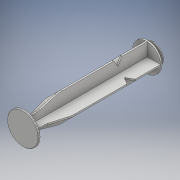
# Autodesk Inventor part: Jeringa core
Saved by Autodesk Inventor 2018.3 (Build 223284000, 284)
## iProperties
Created: 2019-02-24
Part Number: Jeringa core
Material: Generic
Document SubType Name: Modeling
Designer: Mario
Density: 1 g/cm^3
Appearance: Default
Author: Mario
Autodesk Inventor part; units mm, degrees
sketch "Sketch1" plane through (0, 0, 0) normal (0, 1, 0) x (-1, 0, 0)
  line L0 (0.75, 0.75) -> (13.75, 0.75)
  line L1 (13.75, 0.75) -> (13.75, -0.75)
  line L2 (13.75, -0.75) -> (0.75, -0.75)
  line L3 (0.75, -0.75) -> (0.75, -13.75)
  line L4 (0.75, -13.75) -> (-0.75, -13.75)
  line L5 (-0.75, -13.75) -> (-0.75, -0.75)
  line L6 (-0.75, -0.75) -> (-13.75, -0.75)
  line L7 (-13.75, -0.75) -> (-13.75, 0.75)
  line L8 (-13.75, 0.75) -> (-0.75, 0.75)
  line L9 (-0.75, 0.75) -> (-0.75, 13.75)
  line L10 (-0.75, 13.75) -> (0.75, 13.75)
  line L11 (0.75, 13.75) -> (0.75, 0.75)
  line L12 (0.75, 0.75) -> (-0.75, -0.75) construction
  line L13 (-0.75, 0.75) -> (0.75, -0.75) construction
  point P0 (0, 0)
  point P1 (0, 0)
  dimension "d0" = 1.5
  dimension "d24" = 27.5
  constraints: 28 end point, 10 perpendicular, 5 equal length, 5 point on line, 1 coincident, 1 midpoint, 1 vertical
  measures "d0" distance of L6.end L7.end
  measures "d24" distance between parallel lines of L7 L1
extrude "Extrusion1" add sketch "Sketch1" along normal blind 25
sketch "Sketch2" plane through (0, 25, 0) normal (0, 1, 0) x (1, 0, 0)
  circle A0 centre (0, 0) radius 13.75
  dimension "d4" = 27.5
  constraints: 1 centre point, 1 coincident
  measures "d4" diameter of A0
extrude "Extrusion2" add sketch "Sketch2" along normal blind 1.5
sketch "Sketch3" plane through (0, 26.5, 0) normal (0, 1, 0) x (1, 0, 0)
  line L0 (-0.75, -0.75) -> (-7.25, -0.75)
  line L1 (-0.75, -0.75) -> (-13.75, -0.75) projected
  line L2 (-7.25, 0.75) -> (-0.75, 0.75)
  line L3 (0.75, 0.75) -> (7.25, 0.75)
  line L4 (0.75, 0.75) -> (13.75, 0.75) projected
  line L5 (7.25, 0.75) -> (7.25, -0.75)
  line L6 (7.25, -0.75) -> (0.75, -0.75)
  line L7 (0.75, -0.75) -> (0.75, -7.75)
  line L8 (0.75, -7.75) -> (-0.75, -7.75)
  line L9 (-0.75, -13.75) -> (-0.75, -0.75) projected
  line L10 (-0.75, -7.75) -> (-0.75, -0.75)
  line L11 (-0.75, -0.75) -> (-0.75, 0.75)
  line L12 (-0.75, 7.75) -> (0.75, 7.75)
  line L13 (0.75, 7.75) -> (0.75, 0.75)
  line L14 (-0.75, 0.75) -> (-0.75, 13.75) projected
  line L15 (-0.75, 0.75) -> (-0.75, 7.75)
  line L16 (-7.25, 0.75) -> (-7.25, -0.75)
  dimension "d48" = 15.5
  constraints: 26 end point, 6 perpendicular, 2 collinear, 2 equal length, 2 midpoint, 2 point on line, 1 horizontal, 1 parallel, 1 vertical
  measures "d48" distance between parallel lines of L12 L8
extrude "Extrusion3" add sketch "Sketch3" along normal blind 4
sketch "Sketch4" plane through (0, 30.5, 0) normal (0, 1, 0) x (1, 0, 0)
  circle A0 centre (0, 0) radius 13.75 construction
  arc A1 (13.72953, 0.75) -> (0.75, 13.72953) centre (0, 0) ccw construction
  arc A2 (13.72953, -0.75) -> (13.75, 0) centre (0, 0) ccw
  arc A3 (13.75, 0) -> (13.72953, 0.75) centre (0, 0) ccw
  arc A4 (0.75, 13.72953) -> (0, 13.75) centre (0, 0) ccw construction
  arc A5 (0, 13.75) -> (-0.75, 13.72953) centre (0, 0) ccw
  arc A6 (-0.75, 13.72953) -> (-13.72953, 0.75) centre (0, 0) ccw construction
  arc A7 (-13.72953, 0.75) -> (-13.75, 0) centre (0, 0) ccw construction
  arc A8 (-13.75, 0) -> (-13.72953, -0.75) centre (0, 0) ccw construction
  arc A9 (-13.72953, -0.75) -> (-0.75, -13.72953) centre (0, 0) ccw construction
  arc A10 (-0.75, -13.72953) -> (0, -13.75) centre (0, 0) ccw construction
  arc A11 (0, -13.75) -> (0.75, -13.72953) centre (0, 0) ccw construction
  arc A12 (0.75, -13.72953) -> (13.72953, -0.75) centre (0, 0) ccw construction
  circle A13 centre (0, 0) radius 10.25
  dimension "d50" = 20.5
  constraints: 1 centre point, 1 coincident
  measures "d50" diameter of A13
extrude "Extrusion4" add sketch "Sketch4" along normal blind 1
ref_plane "Work Plane1" through (0, -4, 0) normal (0, -1, 0) x (1, 0, 0)
sketch "Sketch6" plane through (0, -4, 0) normal (0, -1, 0) x (1, 0, 0)
  line L0 (0.75, 0.75) -> (6.75, 0.75)
  line L1 (0.75, -0.75) -> (6.75, -0.75)
  line L2 (6.75, 0.75) -> (6.75, -0.75)
  line L3 (0.75, -0.75) -> (0.75, -6.75)
  line L4 (0.75, -6.75) -> (-0.75, -6.75)
  line L5 (-0.75, -6.75) -> (-0.75, -0.75)
  line L6 (-0.75, -0.75) -> (-6.75, -0.75)
  line L7 (-6.75, -0.75) -> (-6.75, 0.75)
  line L8 (-6.75, 0.75) -> (-0.75, 0.75)
  line L9 (-0.75, 0.75) -> (-0.75, 6.75)
  line L10 (-0.75, 6.75) -> (0.75, 6.75)
  line L11 (0.75, 6.75) -> (0.75, 0.75)
  point P0 (0, 0)
  dimension "d17" = 13.5
  constraints: 24 end point, 7 perpendicular, 3 equal length, 2 point on line, 2 vertical, 1 horizontal, 1 parallel
  measures "d17" distance of L0.end L7.end
loft "Loft1" add profiles "Sketch6" section 1 edges at (-7.25, 0, 0.75) (-13.75, 0, 0) (-7.25, 0, -0.75) (-0.75, 0, -7.25) (0, 0, -13.75) (0.75, 0, -7.25) (7.25, 0, -0.75) (13.75, 0, 0) (7.25, 0, 0.75) (0.75, 0, 7.25) (0, 0, 13.75) (-0.75, 0, 7.25)
ref_plane "Work Plane2" through (-6.75, -8, 0.75) normal (0, -1, 0) x (1, 0, 0)
sketch "Sketch7" plane through (-6.75, -8, 0.75) normal (0, -1, 0) x (1, 0, 0)
  line L0 (7.5, 0) -> (20.47953, 0)
  line L1 (7.5, 0) -> (13.5, 0)
  line L2 (20.5, 0) -> (13.5, 0)
  line L3 (-6.97953, 0) -> (6, 0)
  line L4 (-7, 0) -> (0, 0)
  line L5 (0, 0) -> (6, 0)
  line L6 (6, 0) -> (6, 12.97953)
  line L7 (6, 0) -> (6, 6)
  line L8 (6, 13) -> (6, 6)
  line L9 (6, -14.47953) -> (6, -1.5)
  line L10 (6, -14.5) -> (6, -7.5)
  line L11 (6, -7.5) -> (6, -1.5)
  line L12 (7.5, 12.97953) -> (7.5, 0)
  line L13 (7.5, 13) -> (7.5, 6)
  line L14 (7.5, 6) -> (7.5, 0)
  line L15 (7.5, -1.5) -> (7.5, -14.47953)
  line L16 (7.5, -1.5) -> (7.5, -7.5)
  line L17 (7.5, -14.5) -> (7.5, -7.5)
  line L18 (20.5, -1.5) -> (20.5, 0)
  line L19 (7.5, 13) -> (6, 13)
  line L20 (-7, 0) -> (-7, -1.5)
  line L21 (6, -1.5) -> (-6.97953, -1.5)
  line L22 (6, -1.5) -> (0, -1.5)
  line L23 (-7, -1.5) -> (0, -1.5)
  line L24 (20.5, 0) -> (7.5, 0)
  line L25 (20.47953, -1.5) -> (7.5, -1.5)
  line L26 (20.5, -1.5) -> (13.5, -1.5)
  line L27 (13.5, -1.5) -> (7.5, -1.5)
  line L28 (6, -14.5) -> (7.5, -14.5)
  line L29 (6, -14.5) -> (6, -1.5)
  line L30 (-7, -1.5) -> (-7, 0)
  line L31 (-7, 0) -> (6, 0)
  line L32 (6, 13) -> (7.5, 13)
  line L33 (7.5, 0) -> (20.5, 0)
  line L34 (20.5, 0) -> (20.5, -1.5)
  line L35 (13.5, -1.5) -> (7.5, -1.5)
  line L36 (7.5, -1.5) -> (20.5, -1.5)
  line L37 (7.5, -14.5) -> (7.5, -1.5)
  line L38 (7.5, 0) -> (7.5, 13)
  line L39 (7.5, -14.5) -> (6, -14.5)
  line L40 (-7, -1.5) -> (6, -1.5)
  line L41 (6, 0) -> (6, 13)
  line L42 (6.75, -14.5) -> (6, -14.5)
  line L43 (7.5, -14.5) -> (6.75, -14.5)
  line L44 (20.5, -1.5) -> (20.47953, -1.5)
  line L45 (-6.97953, -1.5) -> (-7, -1.5)
  line L46 (-7, -0.75) -> (-7, 0)
  line L47 (-7, -1.5) -> (-7, -0.75)
  line L48 (6.75, 13) -> (7.5, 13)
  line L49 (6, 13) -> (6.75, 13)
  line L50 (20.5, -0.75) -> (20.5, -1.5)
  line L51 (20.5, 0) -> (20.5, -0.75)
  line L52 (7.5, -14.47953) -> (7.5, -14.5)
  line L53 (7.5, 13) -> (7.5, 12.97953)
  line L54 (6, -14.5) -> (6, -14.47953)
  line L55 (6, 12.97953) -> (6, 13)
  line L56 (-7, 0) -> (-6.97953, 0)
  line L57 (20.47953, 0) -> (20.5, 0)
  point P0 (6.75, -0.75)
  constraints: 24 end point, 5 perpendicular, 3 collinear, 2 parallel, 2 vertical, 2 other
sketch "Sketch7 outline for Loft2" plane through (-6.75, -8, 0.75) normal (0, -1, 0) x (1, 0, 0)
  line L0 (20.5, -1.5) -> (20.5, 0)
  line L1 (7.5, -1.5) -> (20.5, -1.5)
  line L2 (7.5, -14.5) -> (7.5, -1.5)
  line L3 (6, -14.5) -> (7.5, -14.5)
  line L4 (6, -1.5) -> (6, -14.5)
  line L5 (-7, -1.5) -> (6, -1.5)
  line L6 (-7, 0) -> (-7, -1.5)
  line L7 (6, 0) -> (-7, 0)
  line L8 (6, 13) -> (6, 0)
  line L9 (7.5, 13) -> (6, 13)
  line L10 (7.5, 0) -> (7.5, 13)
  line L11 (20.5, 0) -> (7.5, 0)
loft "Loft2" add profiles "Sketch7 outline for Loft2" section 1 edges at (-3.75, -4, 0.75) (-6.75, -4, 0) (-3.75, -4, -0.75) (-0.75, -4, -3.75) (0, -4, -6.75) (0.75, -4, -3.75) (3.75, -4, -0.75) (6.75, -4, 0) (3.75, -4, 0.75) (0.75, -4, 3.75) (0, -4, 6.75) (-0.75, -4, 3.75)
fillet "Fillet1" radius 0.5 8 edges at (0, -4, 6.75) (0, 0, 13.75) (-6.75, -4, 0) (-13.75, 0, 0) (0, -4, -6.75) (0, 0, -13.75) (6.75, -4, 0) (13.75, 0, 0)
sketch "Sketch8" plane through (-13.75, -8, -0.75) normal (0, -1, 0) x (1, 0, 0)
  line L0 (0, 1.5) -> (0, 0) projected
  line L1 (0, 0) -> (13, 0) projected
  line L2 (13, 0) -> (13, -13) projected
  line L3 (13, -13) -> (14.5, -13) projected
  line L4 (14.5, -13) -> (14.5, 0) projected
  line L5 (14.5, 0) -> (27.5, 0) projected
  line L6 (27.5, 0) -> (27.5, 1.5) projected
  line L7 (27.5, 1.5) -> (14.5, 1.5) projected
  line L8 (14.5, 1.5) -> (14.5, 14.5) projected
  line L9 (14.5, 14.5) -> (13, 14.5) projected
  line L10 (13, 14.5) -> (13, 1.5) projected
  line L11 (13, 1.5) -> (0, 1.5) projected
  point P0 (13.75, 0.75)
extrude "Extrusion5" add sketch "Sketch8" along normal blind 54
fillet "Fillet2" radius 0.5 4 edges at (0, -8, 13.75) (13.75, -8, 0) (0, -8, -13.75) (-13.75, -8, 0)
ref_plane "Work Plane3" through (-13.75, -82, -0.75) normal (0, -1, 0) x (1, 0, 0)
sketch "Sketch9" plane through (-13.75, -82, -0.75) normal (0, -1, 0) x (1, 0, 0)
  line L0 (14.5, 1.5) -> (21.75, 1.5)
  line L1 (21.75, 1.5) -> (21.75, 0)
  line L2 (21.75, 0) -> (14.5, 0)
  line L3 (14.5, 0) -> (14.5, -7.25)
  line L4 (14.5, -7.25) -> (13, -7.25)
  line L5 (13, -7.25) -> (13, 0)
  line L6 (13, 0) -> (5.75, 0)
  line L7 (5.75, 0) -> (5.75, 1.5)
  line L8 (5.75, 1.5) -> (13, 1.5)
  line L9 (13, 1.5) -> (13, 8.75)
  line L10 (13, 8.75) -> (14.5, 8.75)
  line L11 (14.5, 8.75) -> (14.5, 1.5)
  point P0 (13.75, 0.75)
  dimension "d29" = 16
  constraints: 24 end point, 7 parallel, 6 equal length, 3 perpendicular
  measures "d29" distance between parallel lines of L4 L10
loft "Loft3" add profiles "Sketch9" section 1 edges at (-13.75, -62, 0) (-7.25, -62, -0.75) (-0.75, -62, -7.25) (0, -62, -13.75) (0.75, -62, -7.25) (7.25, -62, -0.75) (13.75, -62, 0) (7.25, -62, 0.75) (0.75, -62, 7.25) (0, -62, 13.75) (-0.75, -62, 7.25) (-7.25, -62, 0.75)
sketch "Sketch10" plane through (-8, -82, -0.75) normal (0, -1, 0) x (1, 0, 0)
  line L0 (0, 0) -> (0, 1.5) projected
  line L1 (7.25, 0) -> (0, 0) projected
  line L2 (7.25, -7.25) -> (7.25, 0) projected
  line L3 (8.75, -7.25) -> (7.25, -7.25) projected
  line L4 (8.75, 0) -> (8.75, -7.25) projected
  line L5 (16, 0) -> (8.75, 0) projected
  line L6 (16, 1.5) -> (16, 0) projected
  line L7 (8.75, 1.5) -> (16, 1.5) projected
  line L8 (8.75, 8.75) -> (8.75, 1.5) projected
  line L9 (7.25, 8.75) -> (8.75, 8.75) projected
  line L10 (7.25, 1.5) -> (7.25, 8.75) projected
  line L11 (0, 1.5) -> (7.25, 1.5) projected
  point P0 (8, 0.75)
extrude "Extrusion6" add sketch "Sketch10" along normal blind 13
sketch "Sketch11" plane through (-8, -95, -0.75) normal (0, -1, 0) x (1, 0, 0)
  circle A0 centre (8, 0.75) radius 15.5
  dimension "d36" = 31
  constraints: 1 centre point, 1 coincident
  measures "d36" diameter of A0
extrude "Extrusion7" add sketch "Sketch11" along normal blind 2
fillet "Fillet3" radius 0.5 2 edges at (-15.5, -97, 0) (-15.5, -95, 0)
fillet "Fillet4" radius 10 4 edges at (0, -82, -8) (8, -82, 0) (0, -82, 8) (-8, -82, 0)
fillet "Fillet5" radius 20 4 edges at (0, -62, 13.75) (-13.75, -62, 0) (0, -62, -13.75) (13.75, -62, 0)
sketch "Sketch14" plane through (0, 31.5, 0) normal (0, 1, 0) x (1, 0, 0)
  line L0 (-0.75, -0.75) -> (-10, -0.75)
  line L1 (-10, -0.75) -> (-10, 0.75)
  line L2 (-10, 0.75) -> (-0.75, 0.75)
  line L3 (-0.75, 0.75) -> (-0.75, 10)
  line L4 (-0.75, 10) -> (0.75, 10)
  line L5 (0.75, 0.75) -> (0.75, 10)
  line L6 (0.75, 0.75) -> (10, 0.75)
  line L7 (10, -0.75) -> (10, 0.75)
  line L8 (10, -0.75) -> (0.75, -0.75)
  line L9 (0.75, -0.75) -> (0.75, -10)
  line L10 (0.75, -10) -> (-0.75, -10)
  line L11 (-0.75, -10) -> (-0.75, -0.75)
  point P0 (0, 0)
  dimension "d51" = 20
  constraints: 24 end point, 8 perpendicular, 4 equal length, 2 point on line, 1 horizontal, 1 vertical
  measures "d51" distance between parallel lines of L7 L1
extrude "Extrusion8" add sketch "Sketch14" along normal blind 4
sketch "Sketch17" plane through (0, 0, 0) normal (1, 0, 0) x (0, 1, 0)
  line L0 (-123.5, 0) -> (62, 0)
  line L1 (35.5, 0.75) -> (35.5, -0.75)
  line L2 (35.5, 0) -> (35.5, 15)
  line L3 (35.5, 15) -> (30.040446, 15)
  line L4 (30.040446, 15) -> (35.5, 0)
  point P0 (0, 0)
  dimension "d63" = 20
  dimension "d64" = 15
  constraints: 6 end point, 1 midpoint, 1 perpendicular, 1 vertical
  measures "d63" angle of L4 L2
  measures "d64" distance between parallel lines of L0 L3
sketch "Sketch17 outline for Revolution2" plane through (0, 0, 0) normal (1, 0, 0) x (0, 1, 0)
  line L0 (30.040446, 15) -> (35.5, 0)
  line L1 (35.5, 15) -> (30.040446, 15)
  line L2 (35.5, 0) -> (35.5, 15)
revolve "Revolution2" cut sketch "Sketch17 outline for Revolution2" angle 360 about axis through (0, -10, 0) along (0, 1, 0)
body "Solid1"
